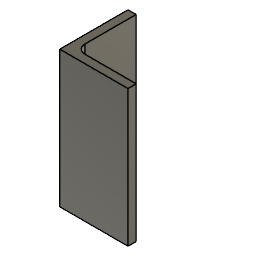
L-50×50×6 (Autodesk Fusion 360 design; units mm, degrees)
Autodesk Fusion 360 part; units mm, degrees
note: some values were not read from the file. Set by a fixed rule: which sketch regions a step uses.
sketch "スケッチ1" plane through (0, 0, 0) normal (0, 0, 1) x (1, 0, 0)
  line L0 (0, 50) -> (0, 0)
  line L1 (50, 6) -> (12.5, 6)
  line L2 (0, 0) -> (50, 0)
  line L3 (6, 12.5) -> (6, 50)
  arc A0 (6, 12.5) -> (12.5, 6) centre (12.5, 12.5) ccw
  line L4 (50, 0) -> (50, 6)
  line L5 (6, 50) -> (0, 50)
extrude "押し出し1" add sketch "スケッチ1" along normal blind 100
